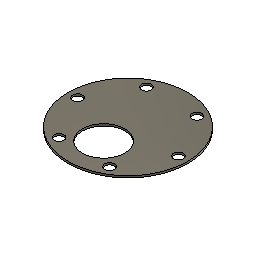
Robot+Mower+3 (Autodesk Fusion 360 archive; units mm, degrees)
design "Motor Template"
Autodesk Fusion 360 part; units mm, degrees
sketch "Sketch1" plane through (0, 0, 0) normal (0, 1, 0) x (1, 0, 0)
  circle A0 centre (0, 0) radius 6.5
  circle A1 centre (0, 7.5) radius 18.375
  line L0 (0, 0) -> (0, 7.5)
  circle A2 centre (0, 7.5) radius 15.5 construction
  line L1 (-26.0681, 7.5) -> (26.0681, 7.5) construction
  circle A3 centre (15.5, 7.5) radius 1.5
  circle A4 centre (7.75, 20.9234) radius 1.5
  circle A5 centre (-7.75, 20.9234) radius 1.5
  circle A6 centre (-15.5, 7.5) radius 1.5
  circle A7 centre (-7.75, -5.9234) radius 1.5
  circle A8 centre (7.75, -5.9234) radius 1.5
  line L2 (-19.977, -10.875) -> (20.9733, -10.875) construction
  dimension "d1" = 13
  dimension "d2" = 36.75
  dimension "d3" = 7.5
  dimension "d4" = 31
  dimension "d5" = 3
  dimension "d7" = 360
  dimension "d10" = 10.875
  constraint coincident A0.centre L0.start
  constraint coincident A1.centre L0.end
  constraint vertical L0
  constraint concentric A1 A2
  constraint horizontal L1
  constraint midpoint A1.centre L1
  constraint coincident A2 A3.centre
  constraint coincident L1 A3.centre
  constraint horizontal L2
  constraint tangent A1 L2
  measures "d1" diameter of A0
  measures "d2" diameter of A1
  measures "d3" distance of A0.centre A1.centre
  measures "d4" diameter of A2
  measures "d5" diameter of A3
  measures "d10" distance of A0.centre L2
extrude "Extrude1" add sketch "Sketch1" along normal blind 0.6
